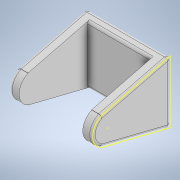
# Autodesk Inventor part: schouder(s)
Saved by Autodesk Inventor 2022 (Build 260153000, 153)
## iProperties
Created: 2022-04-21
Part Number: schouder(s)
Material: Generic
Document SubType Name: Modeling
Designer: kajve
Density: 1 g/cm^3
Appearance: Default
Author: kajve
Autodesk Inventor part; units mm, degrees
ref_plane "YZ Plane" through (0, 0, 0) normal (1, 0, 0) x (0, 1, 0)
ref_plane "XZ Plane" through (0, 0, 0) normal (0, 1, 0) x (-1, 0, 0)
ref_plane "XY Plane" through (0, 0, 0) normal (0, 0, 1) x (1, 0, 0)
sketch "Sketch1" plane through (0, 0, 0) normal (0, 0, 1) x (1, 0, 0)
  point P0 (0, 0)
sketch "Sketch2" plane through (0, 0, 0) normal (0, 0, 1) x (1, 0, 0)
  line L0 (0, 0) -> (60, 0)
  line L1 (60, 0) -> (60, 45)
  line L2 (60, 45) -> (0, 45)
  line L3 (0, 45) -> (0, 0)
  dimension "d0" = 60
  dimension "d1" = 45
  constraints: 8 end point, 2 parallel, 1 horizontal, 1 perpendicular
  measures "d0" distance of L2.end L1.end
  measures "d1" distance of L1.end L0.end
extrude "Extrusion1" add sketch "Sketch2" along normal blind 50
sketch "Sketch3" plane through (60, 0, 0) normal (1, 0, 0) x (0, 0, -1)
  line L0 (0, 45) -> (-50, 45) projected
  line L1 (-50, 0) -> (-50, 45) projected
  line L2 (0, 0) -> (-50, 0) projected
  line L3 (0, 45) -> (-50, 32.5336)
  line L4 (0, 45) -> (51.5307, 45) construction
  line L5 (0, 0) -> (-50, 12.4664)
  line L6 (0, 0) -> (51.5307, 0) construction
  dimension "d4" = 166
  dimension "d5" = 166
  constraints: 8 end point, 2 equal length, 2 horizontal, 2 point on line
  measures "d4" angle of L3 L4
  measures "d5" angle of L6 L5
extrude "Extrusion2" cut sketch "Sketch3" against normal through all
sketch "Sketch4" plane through (60, 0, 0) normal (1, 0, 0) x (0, 0, -1)
  line L0 (-50, 12.4664) -> (-50, 32.5336) projected
  circle A0 centre (-45.6937, 22.5) radius 10.7721
  point P0 (-50, 32.3739)
  point P1 (-50, 12.6261)
  constraints: 1 centre point
extrude "Extrusion3" add sketch "Sketch4" against normal blind 60 contours A0 L0 picked at (-52.7772, 22.9072)
sketch "Sketch6" plane through (0, 0, 0) normal (0, 0, -1) x (-1, 0, 0)
  line L0 (0, 0) -> (-60, 0) projected
  line L1 (-60, 45) -> (0, 45) projected
  line L2 (-7, 0) -> (-53, 0)
  line L3 (-53, 0) -> (-53, 45)
  line L4 (-53, 45) -> (-7, 45)
  line L5 (-7, 45) -> (-7, 0)
  point P0 (-7, 45)
  dimension "d10" = 46
  constraints: 8 end point, 2 parallel, 2 point on line, 1 horizontal, 1 perpendicular
  measures "d10" distance of L3.end L4.end
extrude "Extrusion4" cut sketch "Sketch6" against normal through all
sketch "Sketch7" plane through (0, 0, 0) normal (0, 0, -1) x (-1, 0, 0)
  line L0 (-7, 45) -> (-7, 0) projected
  line L1 (-7, 32.5336) -> (-7, 45) projected
  line L2 (-53, 0) -> (-60, 0) projected
  line L3 (-7, 45) -> (-53, 45)
  line L4 (-53, 45) -> (-53, 0)
  line L5 (-53, 0) -> (-7, 0)
  line L6 (-7, 0) -> (-7, 45)
  point P0 (-7, 0)
  constraints: 8 end point, 2 parallel, 1 horizontal, 1 perpendicular
extrude "Extrusion5" add sketch "Sketch7" against normal blind 7
sketch "Sketch8" plane through (60, 0, 0) normal (1, 0, 0) x (0, 0, -1)
  line L0 (0, 45) -> (-50, 32.5336) projected
  line L1 (-50, 32.3739) -> (-50, 32.5336) projected
  arc A0 (-50, 32.3739) -> (-50, 12.6261) centre (-45.6937, 22.5) ccw projected
  line L2 (-50, 12.4664) -> (-50, 12.6261) projected
  line L3 (-50, 12.4664) -> (0, 0) projected
  line L4 (0, 0) -> (0, 45) projected
sketch "Sketch9" plane through (53, 43.2547, 7) normal (1, 0, 0) x (0, 0, -1)
  line L0 (7, 1.7453) -> (0, 0) projected
  line L1 (7, 1.7453) -> (0, 1.7453) projected
  line L2 (0, 0) -> (0, 1.7453) projected
  line L3 (7, -43.2547) -> (7, 1.7453) projected
  line L4 (0, 0) -> (7, 1.7453)
  line L5 (7, 1.7453) -> (0, 1.7453)
  constraints: 4 end point, 1 collinear
extrude "Extrusion6" cut sketch "Sketch9" against normal through all
sketch "Sketch10" plane through (53, 0, 7) normal (1, 0, 0) x (0, 0, -1)
  line L0 (0, 1.7453) -> (7, 0) projected
  line L1 (0, 0) -> (0, 1.7453) projected
  line L2 (7, 0) -> (0, 0) projected
  line L3 (-43, 12.4664) -> (7, 0) projected
  line L4 (0, 43.2547) -> (0, 1.7453) projected
  line L5 (7, 0) -> (0, 1.7453)
  line L6 (0, 1.7453) -> (0, 0)
  constraints: 4 end point, 1 collinear
extrude "Extrusion7" cut sketch "Sketch10" against normal through all
fillet "Fillet1" radius 2 12 edges at (60, 6.2332, 25) (60, 22.5, 56.4658) (60, 38.7668, 25) (60, 22.5, 0) (30, 0, 0) (30, 45, 0) (0, 22.5, 0) (0, 6.2332, 25) (0, 22.5, 56.4658) (0, 38.7668, 25) (30, 43.2547, 7) (30, 1.7453, 7)
body "Solid1"
